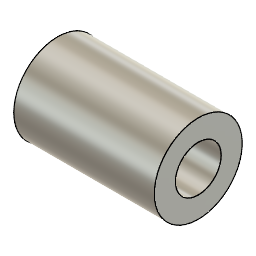
固定盖 (Autodesk Fusion 360 design; units mm, degrees)
part number: 2025-10-23-22-17-23-954
Autodesk Fusion 360 part; units mm, degrees
sketch "草图1" plane through (0, 0, 0) normal (1, 0, 0) x (0, 0, -1)
  circle A0 centre (0, 0) radius 1.3
  circle A1 centre (0, 0) radius 2.5
  dimension "d1" = 2.6
  dimension "d2" = 5
  constraint coincident A0.centre A1.centre
  measures "d1" diameter of A0
  measures "d2" diameter of A1
extrude "拉伸1" add sketch "草图1" along normal blind 8
